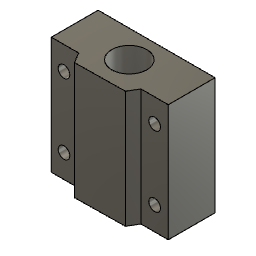
Крепеж для реек v1 (Autodesk Fusion 360 design; units mm, degrees)
Autodesk Fusion 360 part; units mm, degrees
note: some values were not read from the file. Set by a fixed rule: which sketch regions a step uses.
sketch "Sketch1" plane through (0, 0, 0) normal (0, 1, 0) x (1, 0, 0)
  circle A0 centre (0, 0) radius 4.5
  line L0 (15, -18) -> (-15, -18)
  line L1 (-15, -18) -> (-15, 18)
  line L2 (-15, 18) -> (15, 18)
  line L3 (15, 18) -> (15, -18)
  line L4 (15, -18) -> (-15, 18) construction
  line L5 (-15, -18) -> (15, 18) construction
  line L6 (-15, -7) -> (-8, -7)
  line L7 (-8, -7) -> (-6, -10)
  line L8 (-6, -10) -> (6, -10)
  line L9 (6, -10) -> (8, -7)
  line L10 (8, -7) -> (15, -7)
  line L11 (-15, 7) -> (15, 7)
  line L12 (-15, -5) -> (-8, -5)
  line L13 (-8, -5) -> (-5, -10)
  line L14 (5, -10) -> (8, -5)
  line L15 (8, -5) -> (15, -5)
  line L16 (-6.3953, -7.6744) -> (6.5, -7.5)
  dimension "d1" = 9
  constraint coincident A0.centre origin
  constraint horizontal L0
  constraint perpendicular L0 L1
  constraint parallel L0 L2
  constraint parallel L1 L3
  constraint coincident L4 A0.centre
  constraint coincident L5 A0.centre
  constraint coincident L1 L6.start
  constraint perpendicular L1 L6
  constraint parallel L6 L8
  constraint coincident L3 L10.end
  constraint perpendicular L3 L10
  constraint coincident L1 L11.start
  constraint coincident L3 L11.end
  constraint perpendicular L3 L11
  constraint coincident L1 L12.start
  constraint perpendicular L1 L12
  constraint coincident L8 L14.start
  constraint coincident L3 L15.end
  constraint perpendicular L3 L15
  constraint coincident L13 L16.start
  constraint coincident L5 L16.start
  constraint midpoint L14 L16.end
  measures "d1" diameter of A0
extrude "Extrude1" add sketch "Sketch1" along normal blind 30 contours L1 L3 L11 L12 L13 L14 L15 L16
sketch "Sketch2" plane through (0, 0, 5) normal (0, 0, 1) x (1, 0, 0)
  line L0 (8, 0) -> (15, 0)
  line L1 (15, 0) -> (15, 30)
  line L2 (15, 30) -> (8, 30)
  line L3 (8, 30) -> (8, 0)
  line L4 (-11.766, 29.9998) -> (-11.766, -2)
  line L5 (11.5, 30) -> (11.5, -1)
  line L6 (-15, 24) -> (17, 24)
  line L7 (-16, 6) -> (16, 6)
  circle A0 centre (-11.766, 6) radius 1.5
  circle A1 centre (11.5, 6) radius 1.5
  circle A2 centre (11.5, 24) radius 1.5
  circle A3 centre (-11.766, 24) radius 1.5
  dimension "d4" = 3
  dimension "d5" = 3
  dimension "d6" = 3
  dimension "d7" = 3
  constraint parallel L1 L4
  constraint midpoint L2 L5.start
  constraint perpendicular L0 L5
  constraint perpendicular L1 L6
  constraint perpendicular L1 L7
  constraint coincident L4 A0.centre
  constraint coincident L7 A0.centre
  constraint coincident L5 A1.centre
  constraint coincident L7 A1.centre
  constraint coincident L5 A2.centre
  constraint coincident L6 A2.centre
  constraint coincident L4 A3.centre
  constraint coincident L6 A3.centre
  measures "d4" diameter of A0
  measures "d5" diameter of A1
  measures "d6" diameter of A2
  measures "d7" diameter of A3
extrude "Extrude2" cut sketch "Sketch2" against normal blind 14 contours L5 L7 A1 | L5 L7 A1 | L4 L7 A0 | L4 L7 A0 | L5 L7 A1 | L5 L7 A1 | L4 L6 A3 | L4 L6 A3 | L5 L6 A2 | L5 L6 A2 | L4 L7 A0 | L4 L7 A0 | L4 L6 A3 | L4 L6 A3 | L5 L6 A2 | L5 L6 A2
